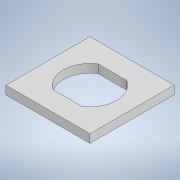
# Autodesk Inventor part: Holes_Test2
Saved by Autodesk Inventor 2022 (Build 260153000, 153)
## iProperties
Created: 2021-07-13
Part Number: Holes_Test2
Material: Generic
Document SubType Name: Modeling
Designer: MJAC
Density: 1 g/cm^3
Appearance: Default
Author: MJAC
Autodesk Inventor part; units mm, degrees
ref_plane "YZ Plane" through (0, 0, 0) normal (1, 0, 0) x (0, 1, 0)
ref_plane "XZ Plane" through (0, 0, 0) normal (0, 1, 0) x (-1, 0, 0)
ref_plane "XY Plane" through (0, 0, 0) normal (0, 0, 1) x (1, 0, 0)
sketch "Sketch1" plane through (0, 0, 0) normal (0, 1, 0) x (-1, 0, 0)
  line L0 (-15, -15) -> (15, -15)
  line L1 (15, -15) -> (15, 15)
  line L2 (15, 15) -> (-15, 15)
  line L3 (-15, 15) -> (-15, -15)
  line L4 (-15, -15) -> (15, 15) construction
  line L5 (15, -15) -> (-15, 15) construction
  point P0 (0, 0)
  dimension "d7" = 30
  dimension "d8" = 30
  constraints: 12 end point, 2 midpoint, 2 parallel, 1 horizontal, 1 perpendicular
  measures "d7" distance of L0.end L1.end
  measures "d8" distance of L1.end L2.end
extrude "Base plate" add sketch "Sketch1" along normal blind 3
sketch "Sketch5" plane through (0, 3, 0) normal (0, 1, 0) x (1, 0, 0)
  circle A0 centre (0, 0) radius 9.5
  line L0 (-15, 15) -> (-15, -15) projected
  line L1 (-15, -15) -> (15, -15) projected
  line L2 (15, 15) -> (-15, 15) projected
  point P0 (0, 0)
  point P1 (8.0777, -15)
  point P2 (-8.0777, -15)
  dimension "d19" = 19
  dimension "d20" = 15
  dimension "d21" = 15
  constraints: 1 centre point
  measures "d19" diameter of A0
  measures "d20" distance from line of L0 A0.centre
  measures "d21" distance from line of L1 A0.centre
extrude "Sleutel 19" cut sketch "Sketch5" against normal through all
sketch "Sketch9" plane through (0, 3, 0) normal (0, 1, 0) x (1, 0, 0)
  line L0 (-9.3784, 15) -> (9.5, 15)
  line L1 (9.5, 15) -> (9.5, 8)
  line L2 (9.5, 8) -> (-9.3784, 8)
  line L3 (-9.3784, 8) -> (-9.3784, 15)
  circle A0 centre (0, 0) radius 9.5 projected
  line L4 (15, 15) -> (-15, 15) projected
  point P0 (0, 0)
  point P1 (-5.1235, 8)
  point P2 (5.1235, 8)
  point P3 (-8.0777, 15)
  point P4 (8.0777, 15)
  dimension "d33" = 8
  dimension "d34" = 0
  constraints: 8 end point, 2 parallel, 1 horizontal, 1 perpendicular, 1 other
  measures "d33" distance from line of point (0, 0) L2
  measures "d34" distance between parallel lines of L4 L0
extrude "Extrusion7" add sketch "Sketch9" against normal up to surface (3 mm away) contours L0 L1 L2 A0 L3 | A0 L2 picked at (-1.0613, 8.3168)
sketch "Sketch10" plane through (0, 3, 0) normal (0, 1, 0) x (1, 0, 0)
  line L0 (-10.3172, -11) -> (10, -11)
  line L1 (10, -11) -> (10, -8)
  line L2 (10, -8) -> (-10.3172, -8)
  line L3 (-10.3172, -8) -> (-10.3172, -11)
  arc A0 (-5.1235, 8) -> (5.1235, 8) centre (0, 0) ccw projected
  point P0 (0, 0)
  point P1 (5.1235, -8)
  point P2 (-5.1235, -8)
  point P3 (-8.0777, 15)
  point P4 (8.0777, 15)
  dimension "d37" = 8
  constraints: 8 end point, 2 parallel, 1 horizontal, 1 perpendicular
  measures "d37" distance from line of A0.centre L2
extrude "Extrusion8" add sketch "Sketch10" against normal up to surface (3 mm away)
body "Solid1"
